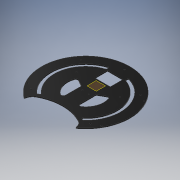
# Autodesk Inventor part: 4th Board
Saved by Autodesk Inventor 2017 (Build 210142000, 142)
## iProperties
Created: 2019-03-15
Part Number: 4th Board
Material: Generic
Document SubType Name: Modeling
Designer: Nicholas Cresswell
Density: 1 g/cm^3
Appearance: Smooth - Black
Author: Nicholas Cresswell
Autodesk Inventor part; units mm, degrees
ref_plane "YZ Plane" through (0, 0, 0) normal (1, 0, 0) x (0, 1, 0)
ref_plane "XZ Plane" through (0, 0, 0) normal (0, 1, 0) x (-1, 0, 0)
ref_plane "XY Plane" through (0, 0, 0) normal (0, 0, 1) x (1, 0, 0)
sketch "Sketch1" plane through (0, 0, 0) normal (0, 0, 1) x (1, 0, 0)
  line L0 (18.5032, 45.3912) -> (18.5032, 14.8912) projected
  line L1 (18.5032, 14.8912) -> (-18.4968, 14.8912) projected
  line L2 (-18.4968, 14.8912) -> (-18.4968, 45.3912) projected
  line L3 (-18.4968, 45.3912) -> (18.5032, 45.3912) projected
  arc A0 (17.5017, -55.6702) -> (25.4619, -59.6998) centre (22.5017, -55.6702) ccw projected
  line L4 (17.5017, -55.6702) -> (17.5016, -25.0441) projected
  arc A1 (17.5016, -25.0441) -> (17.2066, -21.8442) centre (0.0033, -25.0441) ccw projected
  arc A2 (19.6222, -16.5997) -> (17.2066, -21.8442) centre (22.1222, -20.9298) ccw projected
  line L5 (19.6222, -16.5997) -> (33.5153, -8.5785) projected
  arc A3 (40.7535, -11.3119) -> (33.5153, -8.5785) centre (36.0153, -12.9086) ccw projected
  arc A4 (25.4619, -59.6998) -> (40.7535, -11.3119) centre (0.0033, -25.0441) ccw projected
  arc A5 (-17.2054, -21.8447) -> (-19.6211, -16.6006) centre (-22.1212, -20.9307) ccw projected
  arc A6 (-17.2054, -21.8447) -> (-17.5003, -25.0442) centre (0.0033, -25.0441) ccw projected
  line L6 (-17.5003, -25.0442) -> (-17.5003, -55.6665) projected
  arc A7 (-25.4611, -59.6955) -> (-17.5003, -55.6665) centre (-22.5003, -55.6665) ccw projected
  arc A8 (-40.7482, -11.3157) -> (-25.4611, -59.6955) centre (0.0033, -25.0441) ccw projected
  arc A9 (-33.5098, -8.5818) -> (-40.7482, -11.3157) centre (-36.0099, -12.9119) ccw projected
  line L7 (-33.5098, -8.5818) -> (-19.6211, -16.6006) projected
  line L8 (22.5032, 47.8371) -> (22.5032, 51.6387)
  arc A10 (25.1118, 53.5439) -> (22.5032, 51.6387) centre (24.5032, 51.6387) ccw
  arc A11 (-25.1056, 53.5343) -> (-69.0178, 20.1345) centre (0.0033, -25.0441) ccw projected
  arc A12 (-22.4968, 51.6291) -> (-25.1056, 53.5343) centre (-24.4968, 51.6291) ccw
  line L9 (-22.4968, 51.6291) -> (-22.4968, 47.8394)
  arc A13 (53.5122, -86.077) -> (55.8167, -85.7905) centre (54.4635, -84.3178) ccw
  arc A14 (53.5122, -86.077) -> (50.1516, -84.3322) centre (-0.0002, -185.037) ccw
  arc A15 (-50.1523, -84.3319) -> (-53.5093, -86.0748) centre (-0.0002, -185.037) ccw
  arc A16 (-55.8138, -85.7882) -> (-53.5093, -86.0748) centre (-54.4606, -84.3155) ccw
  arc A17 (-62.339, -109.5339) -> (-60.7504, -108.8306) centre (-61.7453, -108.7292) ccw projected
  arc A18 (-50.0022, -92.7062) -> (-60.7504, -108.8306) centre (-40.1313, -110.9304) ccw projected
  arc A19 (50.001, -92.7085) -> (-50.0022, -92.7062) centre (-0.0027, -185.0388) ccw projected
  arc A20 (60.7494, -108.8311) -> (50.001, -92.7085) centre (40.1315, -110.9322) ccw projected
  arc A21 (60.7494, -108.8311) -> (62.3379, -109.5344) centre (61.7442, -108.7297) ccw projected
  arc A22 (62.3379, -109.5344) -> (-62.339, -109.5339) centre (-0.0002, -25.0416) ccw projected
  arc A23 (49.7154, -81.0462) -> (23.8658, 45.9414) centre (-0.0002, -25.0416) ccw
  arc A24 (-23.8596, 45.9436) -> (-49.7161, -81.046) centre (-0.0002, -25.0416) ccw
  arc A25 (55.661, -85.9197) -> (24.8977, 53.5994) centre (-0.0002, -25.0416) ccw
  arc A26 (-25.052, 53.5506) -> (-55.6938, -85.89) centre (-0.0002, -25.0416) ccw
  arc A27 (-50.1523, -84.3319) -> (-49.7161, -81.046) centre (-51.0439, -82.5417) ccw
  arc A28 (49.7154, -81.0462) -> (50.1516, -84.3322) centre (51.0431, -82.5419) ccw
  arc A29 (22.5032, 47.8371) -> (23.8658, 45.9414) centre (24.5032, 47.8371) ccw
  arc A30 (-23.8596, 45.9436) -> (-22.4968, 47.8394) centre (-24.4968, 47.8394) ccw
  point P0 (0, 0)
  point P1 (22.5032, 46.385)
  point P2 (-22.4968, 46.3872)
  dimension "d31" = 2
  constraints: 34 point on circle, 14 centre point, 8 tangent, 4 end point, 3 equal radius, 2 coincident, 2 point on line
  measures "d31" radius of A27
extrude "Extrusion11" add sketch "Sketch1" along normal blind 2
ref_plane "Work Plane9" through (0, 0, 2) normal (0, 0, 1) x (1, 0, 0)
sketch "Sketch4" plane through (0, 0, 2) normal (0, 0, 1) x (1, 0, 0)
  circle A0 centre (0.0001, -25.0412) radius 10.8 projected
  line L0 (0.0001, -25.0412) -> (-7.4999, -25.0412) construction
  circle A1 centre (-7.4999, -25.0412) radius 1.5
  line L1 (0.0001, -25.0412) -> (7.5001, -25.0412) construction
  circle A2 centre (7.5001, -25.0412) radius 1.5
  point P0 (0, 0)
  dimension "d19" = 7.5
  dimension "d20" = 3
  dimension "d21" = 7.5
  dimension "d22" = 3
  constraints: 4 end point, 3 coincident, 2 centre point, 2 horizontal
  measures "d19" distance of L0.start L0.end
  measures "d20" diameter of A1
  measures "d21" distance of L0.start L1.end
  measures "d22" diameter of A2
extrude "Extrusion7" cut sketch "Sketch4" against normal up to next contours A1 | A2
sketch "Sketch8" plane through (0, 0, 0) normal (0, 0, -1) x (-1, 0, 0)
  circle A0 centre (70.8591, 34.4165) radius 1.5
  circle A1 centre (87.6853, 25.5834) radius 1.5
  circle A2 centre (87.6853, -75.6666) radius 1.5
  circle A3 centre (70.8591, -84.4992) radius 1.5
  circle A4 centre (51.8178, 4.8745) radius 1.5
  circle A5 centre (0, 67.4586) radius 1.5
  circle A6 centre (-70.8591, 34.4165) radius 1.5
  circle A7 centre (-51.8178, 4.8745) radius 1.5
  circle A8 centre (-87.6849, 25.5834) radius 1.5
  circle A9 centre (-87.6849, -75.6666) radius 1.5
  circle A10 centre (-70.8591, -84.4992) radius 1.5
  point P0 (0, 0)
  constraints: 11 centre point, 22 other
extrude "Extrusion12" cut sketch "Sketch8" against normal blind 2
body "Solid1"
